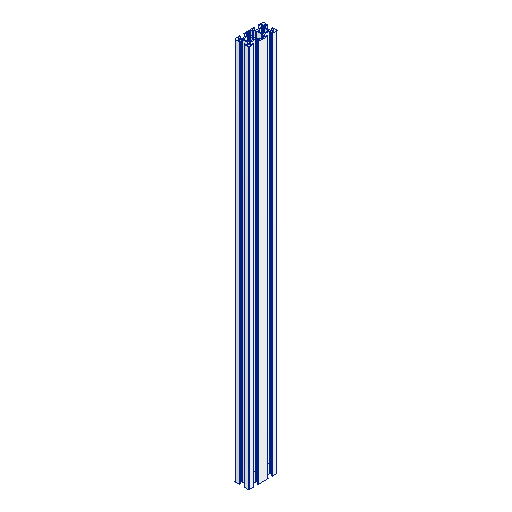
# Autodesk Inventor part: Perfil Viga 1
Saved by Autodesk Inventor 2026.1 (Build 301233000, 233)
## iProperties
Company: Elgin
Created: 2024-10-02
Material: Aluminio 1060
Document SubType Name: Modeling
Density: 2.7 g/cm^3
Appearance: Aluminum - Flat
Description: Perfil Viga 1
Mass: 1336.15 g
Surface Area: 4149.94 cm^2
Volume: 494.872 cm^3
Checked By: Antonio Lucas
Engr Approved By: Antonio Lucas
Mfg Approved By: Anderson Oliveira
Part Number: Perfil Viga 1
Dimensões: 30 x 60 x 800 mm
Total: 4
Author: Willian Pinheiro
Title: Ceteva
Revision Number: 00
Autodesk Inventor part; units mm, degrees
ref_plane "YZ Plane" through (0, 0, 0) normal (1, 0, 0) x (0, 1, 0)
ref_plane "XZ Plane" through (0, 0, 0) normal (0, 1, 0) x (-1, 0, 0)
ref_plane "XY Plane" through (0, 0, 0) normal (0, 0, 1) x (1, 0, 0)
sketch "Sketch1" plane through (0, 0, 0) normal (0, 0, 1) x (1, 0, 0)
  line L0 (0, -31) -> (0, 31) construction
  line L1 (16, 15) -> (-16, 15) construction
  line L2 (16, -15) -> (-16, -15) construction
  arc A0 (-5.7938, 10.2374) -> (-4.7626, 9.2062) centre (0, 15) ccw
  arc A1 (-4.7626, 9.2062) -> (-4.4944, 9.1482) centre (-4.5721, 9.438) ccw
  line L3 (-4.4944, 9.1482) -> (-2.8657, 9.5846)
  arc A2 (-2.6564, 9.5644) -> (-2.8657, 9.5846) centre (-2.7881, 9.2948) ccw
  arc A3 (-2.6564, 9.5644) -> (0, 8.95) centre (0, 15) ccw
  arc A4 (0, 8.95) -> (2.6564, 9.5644) centre (0, 15) ccw
  arc A5 (2.8657, 9.5846) -> (2.6564, 9.5644) centre (2.7881, 9.2948) ccw
  line L4 (2.8657, 9.5846) -> (4.4944, 9.1482)
  arc A6 (4.4944, 9.1482) -> (4.7626, 9.2062) centre (4.5721, 9.438) ccw
  arc A7 (4.7626, 9.2062) -> (5.7938, 10.2374) centre (0, 15) ccw
  arc A8 (5.7938, 10.2374) -> (5.8518, 10.5056) centre (5.562, 10.4279) ccw
  line L5 (5.8518, 10.5056) -> (5.4154, 12.1343)
  arc A9 (5.4356, 12.3436) -> (5.4154, 12.1343) centre (5.7052, 12.2119) ccw
  arc A10 (5.4356, 12.3436) -> (6.05, 15) centre (0, 15) ccw
  arc A11 (6.05, 15) -> (5.4356, 17.6564) centre (0, 15) ccw
  arc A12 (5.4154, 17.8657) -> (5.4356, 17.6564) centre (5.7052, 17.7881) ccw
  line L6 (5.4154, 17.8657) -> (5.8518, 19.4944)
  arc A13 (5.8518, 19.4944) -> (5.7938, 19.7626) centre (5.562, 19.5721) ccw
  arc A14 (5.7938, 19.7626) -> (4.7626, 20.7938) centre (0, 15) ccw
  arc A15 (4.7626, 20.7938) -> (4.4944, 20.8518) centre (4.5721, 20.562) ccw
  line L7 (4.4944, 20.8518) -> (2.8657, 20.4154)
  arc A16 (2.6564, 20.4356) -> (2.8657, 20.4154) centre (2.7881, 20.7052) ccw
  arc A17 (2.6564, 20.4356) -> (0, 21.05) centre (0, 15) ccw
  arc A18 (0, 21.05) -> (-2.6564, 20.4356) centre (0, 15) ccw
  arc A19 (-2.8657, 20.4154) -> (-2.6564, 20.4356) centre (-2.7881, 20.7052) ccw
  line L8 (-2.8657, 20.4154) -> (-4.4944, 20.8518)
  arc A20 (-4.4944, 20.8518) -> (-4.7626, 20.7938) centre (-4.5721, 20.562) ccw
  arc A21 (-4.7626, 20.7938) -> (-5.7938, 19.7626) centre (0, 15) ccw
  arc A22 (-5.7938, 19.7626) -> (-5.8518, 19.4944) centre (-5.562, 19.5721) ccw
  line L9 (-5.8518, 19.4944) -> (-5.4154, 17.8657)
  arc A23 (-5.4356, 17.6564) -> (-5.4154, 17.8657) centre (-5.7052, 17.7881) ccw
  arc A24 (-5.4356, 17.6564) -> (-6.05, 15) centre (0, 15) ccw
  arc A25 (-6.05, 15) -> (-5.4356, 12.3436) centre (0, 15) ccw
  arc A26 (-5.4154, 12.1343) -> (-5.4356, 12.3436) centre (-5.7052, 12.2119) ccw
  line L10 (-5.4154, 12.1343) -> (-5.8518, 10.5056)
  arc A27 (-5.8518, 10.5056) -> (-5.7938, 10.2374) centre (-5.562, 10.4279) ccw
  arc A28 (-4.7626, -9.2062) -> (-5.7938, -10.2374) centre (0, -15) ccw
  arc A29 (-4.4944, -9.1482) -> (-4.7626, -9.2062) centre (-4.5721, -9.438) ccw
  line L11 (-4.4944, -9.1482) -> (-2.8657, -9.5846)
  arc A30 (-2.8657, -9.5846) -> (-2.6564, -9.5644) centre (-2.7881, -9.2948) ccw
  arc A31 (0, -8.95) -> (-2.6564, -9.5644) centre (0, -15) ccw
  arc A32 (2.6564, -9.5644) -> (0, -8.95) centre (0, -15) ccw
  arc A33 (2.6564, -9.5644) -> (2.8657, -9.5846) centre (2.7881, -9.2948) ccw
  line L12 (2.8657, -9.5846) -> (4.4944, -9.1482)
  arc A34 (4.7626, -9.2062) -> (4.4944, -9.1482) centre (4.5721, -9.438) ccw
  arc A35 (5.7938, -10.2374) -> (4.7626, -9.2062) centre (0, -15) ccw
  arc A36 (5.8518, -10.5056) -> (5.7938, -10.2374) centre (5.562, -10.4279) ccw
  line L13 (5.8518, -10.5056) -> (5.4154, -12.1343)
  arc A37 (5.4154, -12.1343) -> (5.4356, -12.3436) centre (5.7052, -12.2119) ccw
  arc A38 (6.05, -15) -> (5.4356, -12.3436) centre (0, -15) ccw
  arc A39 (5.4356, -17.6564) -> (6.05, -15) centre (0, -15) ccw
  arc A40 (5.4356, -17.6564) -> (5.4154, -17.8657) centre (5.7052, -17.7881) ccw
  line L14 (5.4154, -17.8657) -> (5.8518, -19.4944)
  arc A41 (5.7938, -19.7626) -> (5.8518, -19.4944) centre (5.562, -19.5721) ccw
  arc A42 (4.7626, -20.7938) -> (5.7938, -19.7626) centre (0, -15) ccw
  arc A43 (4.4944, -20.8518) -> (4.7626, -20.7938) centre (4.5721, -20.562) ccw
  line L15 (4.4944, -20.8518) -> (2.8657, -20.4154)
  arc A44 (2.8657, -20.4154) -> (2.6564, -20.4356) centre (2.7881, -20.7052) ccw
  arc A45 (0, -21.05) -> (2.6564, -20.4356) centre (0, -15) ccw
  arc A46 (-2.6564, -20.4356) -> (0, -21.05) centre (0, -15) ccw
  arc A47 (-2.6564, -20.4356) -> (-2.8657, -20.4154) centre (-2.7881, -20.7052) ccw
  line L16 (-2.8657, -20.4154) -> (-4.4944, -20.8518)
  arc A48 (-4.7626, -20.7938) -> (-4.4944, -20.8518) centre (-4.5721, -20.562) ccw
  arc A49 (-5.7938, -19.7626) -> (-4.7626, -20.7938) centre (0, -15) ccw
  arc A50 (-5.8518, -19.4944) -> (-5.7938, -19.7626) centre (-5.562, -19.5721) ccw
  line L17 (-5.8518, -19.4944) -> (-5.4154, -17.8657)
  arc A51 (-5.4154, -17.8657) -> (-5.4356, -17.6564) centre (-5.7052, -17.7881) ccw
  arc A52 (-6.05, -15) -> (-5.4356, -17.6564) centre (0, -15) ccw
  arc A53 (-5.4356, -12.3436) -> (-6.05, -15) centre (0, -15) ccw
  arc A54 (-5.4356, -12.3436) -> (-5.4154, -12.1343) centre (-5.7052, -12.2119) ccw
  line L18 (-5.4154, -12.1343) -> (-5.8518, -10.5056)
  arc A55 (-5.7938, -10.2374) -> (-5.8518, -10.5056) centre (-5.562, -10.4279) ccw
  arc A56 (-13, -19.25) -> (-13.1, -19.15) centre (-13.1, -19.25) ccw
  line L19 (-13, -19.25) -> (-13, -24)
  arc A57 (-13, -24) -> (-12.5, -24.5) centre (-12.5, -24) ccw
  line L20 (-12.5, -24.5) -> (-11.1799, -24.5)
  arc A58 (-11.1799, -24.5) -> (-10.9678, -24.4121) centre (-11.1799, -24.2) ccw
  line L21 (-10.9678, -24.4121) -> (-8.7787, -22.223)
  arc A59 (-8.7787, -22.223) -> (-7.9, -20.1017) centre (-10.9, -20.1017) ccw
  line L22 (-7.9, -20.1017) -> (-7.9, -15)
  line L23 (-7.9, -15) -> (-7.9, -9.8983)
  arc A60 (-7.9, -9.8983) -> (-8.7787, -7.777) centre (-10.9, -9.8983) ccw
  line L24 (-8.7787, -7.777) -> (-10.9678, -5.5879)
  arc A61 (-10.9678, -5.5879) -> (-11.1799, -5.5) centre (-11.1799, -5.8) ccw
  line L25 (-11.1799, -5.5) -> (-12.5, -5.5)
  arc A62 (-12.5, -5.5) -> (-13, -6) centre (-12.5, -6) ccw
  line L26 (-13, -6) -> (-13, -10.75)
  arc A63 (-13.1, -10.85) -> (-13, -10.75) centre (-13.1, -10.75) ccw
  line L27 (-13.1, -10.85) -> (-14, -10.85)
  arc A64 (-15, -9.85) -> (-14, -10.85) centre (-14, -9.85) ccw
  line L28 (-15, -9.85) -> (-15, 9.85)
  arc A65 (-14, 10.85) -> (-15, 9.85) centre (-14, 9.85) ccw
  line L29 (-14, 10.85) -> (-13.1, 10.85)
  arc A66 (-13, 10.75) -> (-13.1, 10.85) centre (-13.1, 10.75) ccw
  line L30 (-13, 10.75) -> (-13, 6)
  arc A67 (-13, 6) -> (-12.5, 5.5) centre (-12.5, 6) ccw
  line L31 (-12.5, 5.5) -> (-11.1799, 5.5)
  arc A68 (-11.1799, 5.5) -> (-10.9678, 5.5879) centre (-11.1799, 5.8) ccw
  line L32 (-10.9678, 5.5879) -> (-8.7787, 7.777)
  arc A69 (-8.7787, 7.777) -> (-7.9, 9.8983) centre (-10.9, 9.8983) ccw
  line L33 (-7.9, 9.8983) -> (-7.9, 15)
  line L34 (-7.9, 15) -> (-7.9, 20.1017)
  arc A70 (-7.9, 20.1017) -> (-8.7787, 22.223) centre (-10.9, 20.1017) ccw
  line L35 (-8.7787, 22.223) -> (-10.9678, 24.4121)
  arc A71 (-10.9678, 24.4121) -> (-11.1799, 24.5) centre (-11.1799, 24.2) ccw
  line L36 (-11.1799, 24.5) -> (-12.5, 24.5)
  arc A72 (-12.5, 24.5) -> (-13, 24) centre (-12.5, 24) ccw
  line L37 (-13, 24) -> (-13, 19.25)
  arc A73 (-13.1, 19.15) -> (-13, 19.25) centre (-13.1, 19.25) ccw
  line L38 (-13.1, 19.15) -> (-14, 19.15)
  arc A74 (-15, 20.15) -> (-14, 19.15) centre (-14, 20.15) ccw
  line L39 (-15, 20.15) -> (-15, 28.5)
  arc A75 (-13.5, 30) -> (-15, 28.5) centre (-13.5, 28.5) ccw
  line L40 (-13.5, 30) -> (-5.15, 30)
  arc A76 (-4.15, 29) -> (-5.15, 30) centre (-5.15, 29) ccw
  line L41 (-4.15, 29) -> (-4.15, 28.1)
  arc A77 (-4.25, 28) -> (-4.15, 28.1) centre (-4.25, 28.1) ccw
  line L42 (-4.25, 28) -> (-9, 28)
  arc A78 (-9, 28) -> (-9.5, 27.5) centre (-9, 27.5) ccw
  line L43 (-9.5, 27.5) -> (-9.5, 26.1799)
  arc A79 (-9.5, 26.1799) -> (-9.4121, 25.9678) centre (-9.2, 26.1799) ccw
  line L44 (-9.4121, 25.9678) -> (-7.223, 23.7787)
  arc A80 (-7.223, 23.7787) -> (-5.1017, 22.9) centre (-5.1017, 25.9) ccw
  line L45 (-5.1017, 22.9) -> (0, 22.9)
  line L46 (0, 22.9) -> (5.1017, 22.9)
  arc A81 (5.1017, 22.9) -> (7.223, 23.7787) centre (5.1017, 25.9) ccw
  line L47 (7.223, 23.7787) -> (9.4121, 25.9678)
  arc A82 (9.4121, 25.9678) -> (9.5, 26.1799) centre (9.2, 26.1799) ccw
  line L48 (9.5, 26.1799) -> (9.5, 27.5)
  arc A83 (9.5, 27.5) -> (9, 28) centre (9, 27.5) ccw
  line L49 (9, 28) -> (4.25, 28)
  arc A84 (4.15, 28.1) -> (4.25, 28) centre (4.25, 28.1) ccw
  line L50 (4.15, 28.1) -> (4.15, 29)
  arc A85 (5.15, 30) -> (4.15, 29) centre (5.15, 29) ccw
  line L51 (5.15, 30) -> (13.5, 30)
  arc A86 (15, 28.5) -> (13.5, 30) centre (13.5, 28.5) ccw
  line L52 (15, 28.5) -> (15, 20.15)
  arc A87 (14, 19.15) -> (15, 20.15) centre (14, 20.15) ccw
  line L53 (14, 19.15) -> (13.1, 19.15)
  arc A88 (13, 19.25) -> (13.1, 19.15) centre (13.1, 19.25) ccw
  line L54 (13, 19.25) -> (13, 24)
  arc A89 (13, 24) -> (12.5, 24.5) centre (12.5, 24) ccw
  line L55 (12.5, 24.5) -> (11.1799, 24.5)
  arc A90 (11.1799, 24.5) -> (10.9678, 24.4121) centre (11.1799, 24.2) ccw
  line L56 (10.9678, 24.4121) -> (8.7787, 22.223)
  arc A91 (8.7787, 22.223) -> (7.9, 20.1017) centre (10.9, 20.1017) ccw
  line L57 (7.9, 20.1017) -> (7.9, 15)
  line L58 (7.9, 15) -> (7.9, 9.8983)
  arc A92 (7.9, 9.8983) -> (8.7787, 7.777) centre (10.9, 9.8983) ccw
  line L59 (8.7787, 7.777) -> (10.9678, 5.5879)
  arc A93 (10.9678, 5.5879) -> (11.1799, 5.5) centre (11.1799, 5.8) ccw
  line L60 (11.1799, 5.5) -> (12.5, 5.5)
  arc A94 (12.5, 5.5) -> (13, 6) centre (12.5, 6) ccw
  line L61 (13, 6) -> (13, 10.75)
  arc A95 (13.1, 10.85) -> (13, 10.75) centre (13.1, 10.75) ccw
  line L62 (13.1, 10.85) -> (14, 10.85)
  arc A96 (15, 9.85) -> (14, 10.85) centre (14, 9.85) ccw
  line L63 (15, 9.85) -> (15, -9.85)
  arc A97 (14, -10.85) -> (15, -9.85) centre (14, -9.85) ccw
  line L64 (14, -10.85) -> (13.1, -10.85)
  arc A98 (13, -10.75) -> (13.1, -10.85) centre (13.1, -10.75) ccw
  line L65 (13, -10.75) -> (13, -6)
  arc A99 (13, -6) -> (12.5, -5.5) centre (12.5, -6) ccw
  line L66 (12.5, -5.5) -> (11.1799, -5.5)
  arc A100 (11.1799, -5.5) -> (10.9678, -5.5879) centre (11.1799, -5.8) ccw
  line L67 (10.9678, -5.5879) -> (8.7787, -7.777)
  arc A101 (8.7787, -7.777) -> (7.9, -9.8983) centre (10.9, -9.8983) ccw
  line L68 (7.9, -9.8983) -> (7.9, -15)
  line L69 (7.9, -15) -> (7.9, -20.1017)
  arc A102 (7.9, -20.1017) -> (8.7787, -22.223) centre (10.9, -20.1017) ccw
  line L70 (8.7787, -22.223) -> (10.9678, -24.4121)
  arc A103 (10.9678, -24.4121) -> (11.1799, -24.5) centre (11.1799, -24.2) ccw
  line L71 (11.1799, -24.5) -> (12.5, -24.5)
  arc A104 (12.5, -24.5) -> (13, -24) centre (12.5, -24) ccw
  line L72 (13, -24) -> (13, -19.25)
  arc A105 (13.1, -19.15) -> (13, -19.25) centre (13.1, -19.25) ccw
  line L73 (13.1, -19.15) -> (14, -19.15)
  arc A106 (15, -20.15) -> (14, -19.15) centre (14, -20.15) ccw
  line L74 (15, -20.15) -> (15, -28.5)
  arc A107 (13.5, -30) -> (15, -28.5) centre (13.5, -28.5) ccw
  line L75 (13.5, -30) -> (5.15, -30)
  arc A108 (4.15, -29) -> (5.15, -30) centre (5.15, -29) ccw
  line L76 (4.15, -29) -> (4.15, -28.1)
  arc A109 (4.25, -28) -> (4.15, -28.1) centre (4.25, -28.1) ccw
  line L77 (4.25, -28) -> (9, -28)
  arc A110 (9, -28) -> (9.5, -27.5) centre (9, -27.5) ccw
  line L78 (9.5, -27.5) -> (9.5, -26.1799)
  arc A111 (9.5, -26.1799) -> (9.4121, -25.9678) centre (9.2, -26.1799) ccw
  line L79 (9.4121, -25.9678) -> (7.223, -23.7787)
  arc A112 (7.223, -23.7787) -> (5.1017, -22.9) centre (5.1017, -25.9) ccw
  line L80 (5.1017, -22.9) -> (0, -22.9)
  line L81 (0, -22.9) -> (-5.1017, -22.9)
  arc A113 (-5.1017, -22.9) -> (-7.223, -23.7787) centre (-5.1017, -25.9) ccw
  line L82 (-7.223, -23.7787) -> (-9.4121, -25.9678)
  arc A114 (-9.4121, -25.9678) -> (-9.5, -26.1799) centre (-9.2, -26.1799) ccw
  line L83 (-9.5, -26.1799) -> (-9.5, -27.5)
  arc A115 (-9.5, -27.5) -> (-9, -28) centre (-9, -27.5) ccw
  line L84 (-9, -28) -> (-4.25, -28)
  arc A116 (-4.15, -28.1) -> (-4.25, -28) centre (-4.25, -28.1) ccw
  line L85 (-4.15, -28.1) -> (-4.15, -29)
  arc A117 (-5.15, -30) -> (-4.15, -29) centre (-5.15, -29) ccw
  line L86 (-5.15, -30) -> (-13.5, -30)
  arc A118 (-15, -28.5) -> (-13.5, -30) centre (-13.5, -28.5) ccw
  line L87 (-15, -28.5) -> (-15, -20.15)
  arc A119 (-14, -19.15) -> (-15, -20.15) centre (-14, -20.15) ccw
  line L88 (-14, -19.15) -> (-13.1, -19.15)
  line L89 (-11.5, -3.3) -> (-10.7657, -3.3)
  arc A120 (-9.705, -3.7393) -> (-10.7657, -3.3) centre (-10.7657, -4.8) ccw
  line L90 (-9.705, -3.7393) -> (-7.223, -6.2213)
  arc A121 (-7.223, -6.2213) -> (-5.1017, -7.1) centre (-5.1017, -4.1) ccw
  line L91 (-5.1017, -7.1) -> (0, -7.1)
  line L92 (0, -7.1) -> (5.1017, -7.1)
  arc A122 (5.1017, -7.1) -> (7.223, -6.2213) centre (5.1017, -4.1) ccw
  line L93 (7.223, -6.2213) -> (9.705, -3.7393)
  arc A123 (10.7657, -3.3) -> (9.705, -3.7393) centre (10.7657, -4.8) ccw
  line L94 (10.7657, -3.3) -> (11.5, -3.3)
  arc A124 (11.5, -3.3) -> (13, -1.8) centre (11.5, -1.8) ccw
  line L95 (13, -1.8) -> (13, 0)
  line L96 (13, 0) -> (13, 1.8)
  arc A125 (13, 1.8) -> (11.5, 3.3) centre (11.5, 1.8) ccw
  line L97 (11.5, 3.3) -> (10.7657, 3.3)
  arc A126 (9.705, 3.7393) -> (10.7657, 3.3) centre (10.7657, 4.8) ccw
  line L98 (9.705, 3.7393) -> (7.223, 6.2213)
  arc A127 (7.223, 6.2213) -> (5.1017, 7.1) centre (5.1017, 4.1) ccw
  line L99 (5.1017, 7.1) -> (0, 7.1)
  line L100 (0, 7.1) -> (-5.1017, 7.1)
  arc A128 (-5.1017, 7.1) -> (-7.223, 6.2213) centre (-5.1017, 4.1) ccw
  line L101 (-7.223, 6.2213) -> (-9.705, 3.7393)
  arc A129 (-10.7657, 3.3) -> (-9.705, 3.7393) centre (-10.7657, 4.8) ccw
  line L102 (-10.7657, 3.3) -> (-11.5, 3.3)
  arc A130 (-11.5, 3.3) -> (-13, 1.8) centre (-11.5, 1.8) ccw
  line L103 (-13, 1.8) -> (-13, 0)
  line L104 (-13, 0) -> (-13, -1.8)
  arc A131 (-13, -1.8) -> (-11.5, -3.3) centre (-11.5, -1.8) ccw
  line L105 (-22.4, 0) -> (22.4, 0) construction
  line L106 (0, -44.3746) -> (0, 49.2473) construction
  point P0 (0, 0)
  point P1 (-5.0347, 35.8728)
  point P2 (0, 0)
  point P3 (-10.7657, 3.3)
  point P4 (-7.223, 6.2213)
  point P5 (5.1017, 7.1)
  point P6 (9.705, 3.7393)
  point P7 (11.5, 3.3)
  point P8 (13, -1.8)
  point P9 (10.7657, -3.3)
  point P10 (7.223, -6.2213)
  point P11 (-5.1017, -7.1)
  point P12 (-9.705, -3.7393)
  point P13 (-13, 1.8)
  point P14 (-13, -19.25)
  point P15 (-13.1, -19.15)
  point P16 (-14, -19.15)
  point P17 (-15, -28.5)
  point P18 (-5.15, -30)
  point P19 (-4.15, -28.1)
  point P20 (-9, -28)
  point P21 (-9.5, -26.1799)
  point P22 (-7.223, -23.7787)
  point P23 (5.1017, -22.9)
  point P24 (9.4121, -25.9678)
  point P25 (9.5, -27.5)
  point P26 (4.25, -28)
  point P27 (4.15, -29)
  point P28 (13.5, -30)
  point P29 (15, -20.15)
  point P30 (13.1, -19.15)
  point P31 (13, -24)
  point P32 (11.1799, -24.5)
  point P33 (8.7787, -22.223)
  point P34 (7.9, -9.8983)
  point P35 (12.5, -5.5)
  point P36 (13, -10.75)
  point P37 (14, -10.85)
  point P38 (15, 9.85)
  point P39 (13.1, 10.85)
  point P40 (13, 6)
  point P41 (11.1799, 5.5)
  point P42 (8.7787, 7.777)
  point P43 (7.9, 20.1017)
  point P44 (10.9678, 24.4121)
  point P45 (12.5, 24.5)
  point P46 (13, 19.25)
  point P47 (14, 19.15)
  point P48 (15, 28.5)
  point P49 (5.15, 30)
  point P50 (4.15, 28.1)
  point P51 (9, 28)
  point P52 (9.5, 26.1799)
  point P53 (7.223, 23.7787)
  point P54 (-5.1017, 22.9)
  point P55 (-9.4121, 25.9678)
  point P56 (-9.5, 27.5)
  point P57 (-4.25, 28)
  point P58 (-4.15, 29)
  point P59 (-13.5, 30)
  point P60 (-15, 20.15)
  point P61 (-13.1, 19.15)
  point P62 (-13, 24)
  point P63 (-11.1799, 24.5)
  point P64 (-8.7787, 22.223)
  point P65 (-7.9, 9.8983)
  point P66 (-10.9678, 5.5879)
  point P67 (-12.5, 5.5)
  point P68 (-13, 10.75)
  point P69 (-14, 10.85)
  point P70 (-15, -9.85)
  point P71 (-13.1, -10.85)
  point P72 (-13, -6)
  point P73 (-11.1799, -5.5)
  point P74 (-8.7787, -7.777)
  point P75 (-7.9, -20.1017)
  point P76 (-10.9678, -24.4121)
  point P77 (-12.5, -24.5)
  point P78 (-2.6564, -9.5644)
  point P79 (0, -8.95)
  point P80 (2.6564, -9.5644)
  point P81 (2.8657, -9.5846)
  point P82 (4.7626, -9.2062)
  point P83 (5.7938, -10.2374)
  point P84 (5.8518, -10.5056)
  point P85 (5.4356, -12.3436)
  point P86 (6.05, -15)
  point P87 (5.4356, -17.6564)
  point P88 (5.4154, -17.8657)
  point P89 (5.7938, -19.7626)
  point P90 (4.7626, -20.7938)
  point P91 (4.4944, -20.8518)
  point P92 (2.6564, -20.4356)
  point P93 (0, -21.05)
  point P94 (-2.6564, -20.4356)
  point P95 (-2.8657, -20.4154)
  point P96 (-4.7626, -20.7938)
  point P97 (-5.7938, -19.7626)
  point P98 (-5.8518, -19.4944)
  point P99 (-5.4356, -17.6564)
  point P100 (-6.05, -15)
  point P101 (-5.4356, -12.3436)
  point P102 (-5.4154, -12.1343)
  point P103 (-5.7938, -10.2374)
  point P104 (-4.7626, -9.2062)
  point P105 (-5.4154, 12.1343)
  point P106 (-5.4356, 12.3436)
  point P107 (-6.05, 15)
  point P108 (-5.4356, 17.6564)
  point P109 (-5.8518, 19.4944)
  point P110 (-5.7938, 19.7626)
  point P111 (-4.7626, 20.7938)
  point P112 (-2.8657, 20.4154)
  point P113 (-2.6564, 20.4356)
  point P114 (0, 21.05)
  point P115 (2.6564, 20.4356)
  point P116 (4.4944, 20.8518)
  point P117 (4.7626, 20.7938)
  point P118 (5.7938, 19.7626)
  point P119 (5.4154, 17.8657)
  point P120 (5.4356, 17.6564)
  point P121 (6.05, 15)
  point P122 (5.4356, 12.3436)
  point P123 (5.8518, 10.5056)
  point P124 (5.7938, 10.2374)
  point P125 (4.7626, 9.2062)
  point P126 (2.8657, 9.5846)
  point P127 (2.6564, 9.5644)
  point P128 (0, 8.95)
  point P129 (-2.6564, 9.5644)
  point P130 (-4.4944, 9.1482)
  point P131 (-4.7626, 9.2062)
  point P132 (-5.7938, 10.2374)
  dimension "d3" = 8.3
  dimension "d7" = 30
  dimension "d9" = 60
  dimension "d13" = 30
  constraints: 264 point on circle, 210 end point, 132 centre point, 1 midpoint, 1 vertical, 2 other
  measures "d3" distance of L38.end L29.start
  measures "d7" distance of A118.start A107.end
  measures "d9" distance of A86.end A107.start
  measures "d13" distance of L2.start L1.start
extrude "Extrusion1" add sketch "Sketch1" along normal mid plane 800
sketch "Esboço2" plane through (-15, -9.85, 400) normal (-1, 0, 0) x (0, 0, 1)
  line L0 (-960, 9.85) -> (160, 9.85) construction
  line L1 (-800, 0) -> (-800, 19.7) construction
  point P0 (-400, 9.85)
  point P1 (-775, -5.15)
  point P2 (-775, 24.85)
  dimension "d18" = 25
  dimension "d19" = 30
  constraints: 1 symmetric about line
  measures "d18" distance from line of L1 point (-775, -5.15)
  measures "d19" distance of point (-775, 24.85) point (-775, -5.15)
hole "Furo1" at (-15, -15, -375) at (-15, 15, -375) direction (1, 0, 0) diameter 15 depth 22
body "Solid1"
